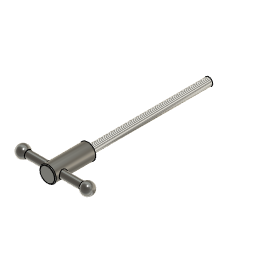
Screw (Autodesk Fusion 360 design; units mm, degrees)
Autodesk Fusion 360 part; units mm, degrees
sketch "Sketch1" plane through (0, 0, 0) normal (0, 1, 0) x (1, 0, 0)
  circle A0 centre (0, 0) radius 25.4
  dimension "d1" = 50.8
  constraint coincident A0.centre origin
  measures "d1" diameter of A0
extrude "Extrude1" add sketch "Sketch1" along normal blind 127 makes body 1
sketch "Sketch3" plane through (0, 0, 0) normal (1, 0, 0) x (0, 1, 0)
  circle A0 centre (25.4, 0) radius 12.7
  dimension "d4" = 25.4
  measures "d4" diameter of A0
extrude "Extrude2" cut sketch "Sketch3" along normal through all and the other way through all bodies 1
sketch "Sketch4" plane through (0, 0, 0) normal (1, 0, 0) x (0, 1, 0)
  circle A0 centre (25.4, 0) radius 11.43
  dimension "d7" = 22.86
  measures "d7" diameter of A0
extrude "Extrude3" add sketch "Sketch4" along normal mid plane 203.2 separate body makes body 2
sphere "SpherePrimitive2" add diameter 38.1 placed x (0, -1, 0) y (0, 0, 1) z (-1, 0, 0) at (-101.6, 25.4, 0) bodies 2
sphere "SpherePrimitive1" add diameter 38.1 placed x (0, 1, 0) y (0, 0, 1) z (1, 0, 0) at (101.6, 25.4, 0) bodies 2
fillet "Fillet1" radius 2.54 1 edges at (-23.6811, 0, 9.185) on bodies 1
sketch "Sketch7" plane through (0, 127, 0) normal (0, 1, 0) x (-1, 0, 0)
  circle A0 centre (0, 0) radius 25.4
  circle A1 centre (0, 0) radius 12.7
  dimension "d14" = 25.4
  constraint coincident A0.centre A1.centre
  measures "d14" diameter of A1
extrude "Extrude4" add sketch "Sketch7" along normal blind 381 contours A1 bodies 1
thread "Thread1" "ANSI Unified Screw Threads 1.0 1-8 UNC 3A" major diameter 25.2095 minor diameter 21.6205 pitch 3.175 angle 60 resizes the face on face at (-12.6369, 381, -1.2645) on bodies 1
